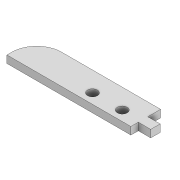
# Autodesk Inventor part: Comb4
Saved by Autodesk Inventor 2020 (Build 240168000, 168)
## iProperties
Created: 2022-04-26
Part Number: Comb4
Material: Generic
Document SubType Name: Modeling
Designer: ferrerx
Density: 1 g/cm^3
Appearance: Default
Author: ferrerx
Autodesk Inventor part; units mm, degrees
ref_plane "YZ Plane" through (0, 0, 0) normal (1, 0, 0) x (0, 1, 0)
ref_plane "XZ Plane" through (0, 0, 0) normal (0, 1, 0) x (-1, 0, 0)
ref_plane "XY Plane" through (0, 0, 0) normal (0, 0, 1) x (1, 0, 0)
sketch "Sketch1" plane through (0, 0, 0) normal (0, 1, 0) x (-1, 0, 0)
  line L0 (25, 100) -> (-25, 100)
  line L1 (-25, 100) -> (-25, -100)
  line L2 (-25, -100) -> (25, -100)
  line L3 (25, -100) -> (25, 100)
  line L4 (25, 100) -> (-25, -100) construction
  line L5 (-25, 100) -> (25, -100) construction
  point P0 (0, 0)
  dimension "d0" = 200
  dimension "d1" = 50
  constraints: 12 end point, 2 midpoint, 2 parallel, 1 horizontal, 1 perpendicular
  measures "d0" distance of L2.end L0.start
  measures "d1" distance of L1.end L2.end
extrude "Extrusion1" add sketch "Sketch1" along normal blind 3
sketch "Sketch2" plane through (0, 3, 0) normal (0, 1, 0) x (1, 0, 0)
  line L0 (0, 0) -> (25, 0) construction
  line L1 (25, -100) -> (25, 100) projected
  line L2 (25, -92) -> (-15.0756, -92) construction
  circle A0 centre (17.5, -92) radius 2
  circle A1 centre (5.5, -92) radius 2
  line L3 (-25, -100) -> (25, -100) projected
  circle A2 centre (17.5, 92) radius 2
  circle A3 centre (5.5, 92) radius 2
  dimension "d4" = 4
  dimension "d5" = 4
  dimension "d6" = 12
  dimension "d7" = 8
  dimension "d10" = 7.5
  constraints: 4 centre point, 4 end point, 3 point on line, 2 symmetric about line, 1 horizontal, 1 midpoint, 2 other
  measures "d4" diameter of A1
  measures "d5" diameter of A0
  measures "d6" distance of A1.centre A0.centre
  measures "d7" distance between parallel lines of L3 L2
  measures "d10" distance from line of L1 A0.centre
extrude "Extrusion2" cut sketch "Sketch2" against normal blind 5
sketch "Sketch3" plane through (0, 3, 0) normal (0, 1, 0) x (1, 0, 0)
  line L0 (19, -85) -> (31, -85)
  line L1 (31, -85) -> (31, 85)
  line L2 (31, 85) -> (19, 85)
  line L3 (19, 85) -> (19, -85)
  line L4 (25, -100) -> (25, 100) projected
  line L5 (19, -85) -> (31, 85) construction
  line L6 (31, -85) -> (19, 85) construction
  point P0 (0, 0)
  point P1 (25, 0)
  dimension "d11" = 170
  dimension "d12" = 12
  constraints: 12 end point, 3 midpoint, 2 parallel, 1 horizontal, 1 perpendicular
  measures "d11" distance of L0.end L1.end
  measures "d12" distance of L1.end L2.end
extrude "Extrusion3" add sketch "Sketch3" against normal blind 3
sketch "Sketch4" plane through (0, 3, 0) normal (0, 1, 0) x (1, 0, 0)
  line L0 (25, -100) -> (25, 100) projected
  line L1 (31, 85) -> (25, 85) projected
  circle A0 centre (26, -75) radius 2
  line L2 (25, -85) -> (31, -85) projected
  line L3 (31, -85) -> (31, 85) projected
  point P0 (0, 0)
  dimension "d15" = 4
  dimension "d16" = 10
  dimension "d17" = 5
  constraints: 1 centre point
  measures "d15" diameter of A0
  measures "d16" distance from line of L2 A0.centre
  measures "d17" distance from line of L3 A0.centre
extrude "Extrusion4" cut sketch "Sketch4" against normal blind 5 contours A0 L0 | L0 A0
pattern_linear "Rectangular Pattern1" count 6 spacing 30 along (0, 0, -1) of "Extrusion4"
fillet "Fillet1" radius 10 2 edges at (-25, 1.5, -100) (-25, 1.5, 100)
sketch "Sketch5" plane through (0, 3, 0) normal (0, 1, 0) x (1, 0, 0)
  line L0 (31, 85) -> (25, 85) projected
  line L1 (32.3908, 88) -> (-29, 88)
  line L2 (-29, 88) -> (-29, -105)
  line L3 (-29, -105) -> (32.3908, -105)
  line L4 (32.3908, -105) -> (32.3908, 84.997)
  line L5 (32.3908, 84.997) -> (32.3908, 88)
  line L6 (25, 100) -> (-15, 100) projected
  point P0 (0, 0)
  dimension "d31" = 12
  constraints: 10 end point, 2 parallel, 1 horizontal, 1 perpendicular, 1 vertical
  measures "d31" distance between parallel lines of L6 L1
extrude "Extrusion5" cut sketch "Sketch5" against normal blind 10
sketch "Sketch6" plane through (0, 3, 0) normal (0, 1, 0) x (1, 0, 0)
  line L0 (25, 94.8) -> (30, 94.8)
  line L1 (30, 94.8) -> (30, 91)
  line L2 (30, 91) -> (25, 91)
  line L3 (25, 91) -> (25, 94.8)
  line L4 (25, 100) -> (-15, 100) projected
  point P0 (0, 0)
  dimension "d26" = 5.2
  dimension "d27" = 5
  dimension "d28" = 3.8
  constraints: 8 end point, 2 parallel, 1 horizontal, 1 perpendicular
  measures "d26" distance between parallel lines of L4 L0
  measures "d27" distance of L1.end L2.end
  measures "d28" distance of L0.end L1.end
extrude "Extrusion6" add sketch "Sketch6" against normal blind 3
body "Solid1"
